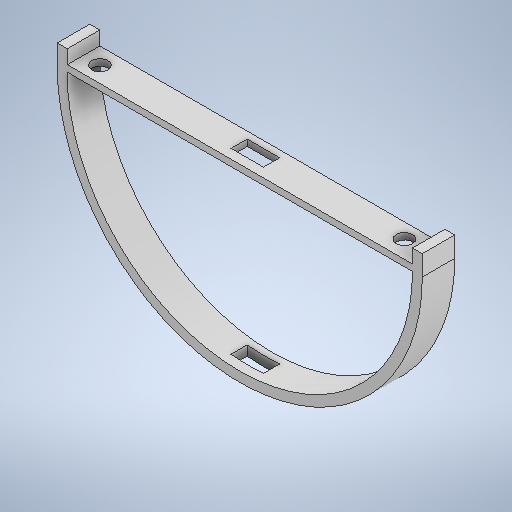
# Autodesk Inventor part: Siding
Saved by Autodesk Inventor 2025 (Build 290162010, 162A)
## iProperties
Created: 2024-06-06
Part Number: Siding
Material: Generic
Document SubType Name: Modeling
Designer: vncnt
Density: 1 g/cm^3
Appearance: Default
Author: vncnt
Autodesk Inventor part; units mm, degrees
ref_plane "YZ Plane" through (0, 0, 0) normal (1, 0, 0) x (0, 1, 0)
ref_plane "XZ Plane" through (0, 0, 0) normal (0, 1, 0) x (-1, 0, 0)
ref_plane "XY Plane" through (0, 0, 0) normal (0, 0, 1) x (1, 0, 0)
sketch "Sketch1" plane through (0, 0, 0) normal (0, 0, 1) x (1, 0, 0)
  arc A0 (-14.2875, 0) -> (14.2875, 0) centre (0, 0) ccw
  arc A1 (-13.5219, 0) -> (13.5219, 0) centre (0, 0) ccw
  line L0 (-14.2875, 0) -> (-13.5219, 0)
  line L1 (13.5219, 0) -> (14.2875, 0)
  constraints: 4 end point, 4 point on circle, 2 centre point, 2 coincident, 2 horizontal
extrude "Extrusion1" add sketch "Sketch1" along normal blind 2.54
sketch "Sketch2" plane through (0, 0, 0) normal (0, 0, -1) x (-1, 0, 0)
  arc A0 (-14.2875, 0) -> (14.2875, 0) centre (0, 0) ccw projected
  line L0 (14.2875, 0) -> (14.2875, 1.5875)
  line L1 (-14.2875, 1.5875) -> (-14.2875, 0)
  line L2 (13.4989, 0.5052) -> (-13.5197, 0.5052)
  line L3 (13.4989, 0.5052) -> (13.4989, 1.5875)
  line L4 (-13.5197, 0.5052) -> (-13.5197, 1.5875)
  line L5 (14.2875, 1.5875) -> (13.4989, 1.5875)
  line L6 (-13.5197, 1.5875) -> (-14.2875, 1.5875)
  line L7 (13.4989, 0) -> (-13.5197, 0)
  line L8 (13.4989, 0) -> (14.2875, 0)
  line L9 (-13.5197, 0) -> (-14.2875, 0)
  constraints: 20 end point, 3 horizontal, 2 perpendicular, 2 vertical, 1 tangent
extrude "Extrusion2" add sketch "Sketch2" against normal blind 2.54 contours L1 L6 L4 L2 L3 L5 L0 L8 L7 L9
sketch "Sketch3" plane through (-13.4989, 0.5052, 0) normal (0, 1, 0) x (1, 0, 0)
  point P0 (13.4989, 0)
  point P1 (1.316, -1.3036)
hole "Hole1" at (-12.1829, 0.5052, 1.3036) direction (0, -1, 0) diameter 1.27 depth 2.54
sketch "Sketch4" plane through (-13.4989, 0.5052, 0) normal (0, 1, 0) x (1, 0, 0)
  point P0 (13.4989, 0)
  point P1 (25.0177, -1.1717)
hole "Hole2" at (11.5188, 0.5052, 1.1717) direction (0, -1, 0) diameter 1.27 depth 2.54
sketch "Sketch5" plane through (-13.4989, 0.5052, 0) normal (0, 1, 0) x (1, 0, 0)
  line L0 (12.0801, -1.8086) -> (14.6201, -1.8086)
  line L1 (14.6201, -1.8086) -> (14.6201, -0.5386)
  line L2 (14.6201, -0.5386) -> (12.0801, -0.5386)
  line L3 (12.0801, -0.5386) -> (12.0801, -1.8086)
  point P0 (13.4989, 0)
  dimension "d18" = 1.27
  dimension "d19" = 2.54
  constraints: 8 end point, 2 parallel, 1 horizontal, 1 perpendicular
  measures "d18" distance of L2.end L0.start
  measures "d19" distance of L0.start L0.end
extrude "Extrusion3" cut sketch "Sketch5" against normal blind 15.24
body "Solid1"
